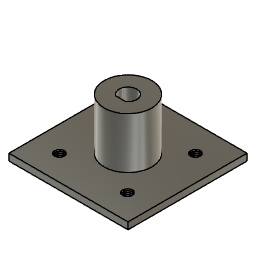
20mm_shaft_extension (Autodesk Fusion 360 design; units mm, degrees)
Autodesk Fusion 360 part; units mm, degrees
sketch "Sketch1" plane through (0, 0, 0) normal (0, 0, 1) x (1, 0, 0)
  line L0 (0, 0) -> (35, 0)
  line L1 (35, 0) -> (35, 35)
  line L2 (35, 35) -> (0, 35)
  line L3 (0, 35) -> (0, 0)
  dimension "d1" = 35
  dimension "d2" = 35
  constraint horizontal L0
  constraint vertical L1
  constraint horizontal L2
  constraint vertical L3
  constraint coincident L0.start L3.end
  measures "d1" distance of L0.start L0.end
  measures "d2" distance of L0.start L2.end
extrude "Extrude1" add sketch "Sketch1" along normal blind 2
sketch "Sketch2" plane through (0, 0, 2) normal (0, 0, 1) x (-1, 0, 0)
  line L0 (0, -35) -> (0, 0)
  line L1 (0, 0) -> (-35, 0)
  line L2 (-35, 0) -> (-35, -35)
  line L3 (-35, -35) -> (0, -35)
  circle A0 centre (-7.5, -27.5) radius 1.5
  circle A1 centre (-27.5, -27.5) radius 1.5
  circle A2 centre (-7.5, -7.5) radius 1.5
  circle A3 centre (-27.5, -7.5) radius 1.5
  dimension "d6" = 3
  dimension "d7" = 3
  dimension "d8" = 3
  dimension "d9" = 3
  dimension "d30" = 20
  dimension "d31" = 20
  dimension "d32" = 20
  dimension "d33" = 20
  dimension "d34" = 7.5
  dimension "d35" = 7.5
  measures "d6" diameter of A0
  measures "d7" diameter of A1
  measures "d8" diameter of A2
  measures "d9" diameter of A3
  measures "d30" distance of A0.centre A1.centre
  measures "d31" distance of A2.centre A3.centre
  measures "d32" distance of A0.centre A2.centre
  measures "d33" distance of A1.centre A3.centre
  measures "d34" distance of L0 A0.centre
  measures "d35" distance of L1 A2.centre
hole "Hole1" at (7.5, 27.5, 2) at (27.5, 27.5, 2) at (27.5, 7.5, 2) at (7.5, 7.5, 2) direction (0, 0, -1) diameter 2.529 depth 2 tip angle 118
thread "Thread1" "ISO Metric profile 3.0 M3x0.5 M3x0.5 6H" major diameter 3.086 minor diameter 2.529 pitch 0.5 angle 60 modelled right hand crest width 0.1368 on face at (27.6259, 6.2418, 1.3333) crest through (28.7645, 7.5, 1.875) on face at (7.6259, 26.2418, 1.3333) crest through (8.7645, 27.5, 1.875) on face at (7.6259, 6.2418, 1.3333) crest through (8.7645, 7.5, 1.875) on face at (27.6259, 26.2418, 1.3333) crest through (28.7645, 27.5, 1.875)
sketch "Sketch3" plane through (0, 0, 2) normal (0, 0, 1) x (-1, 0, 0)
  spline S0 degree 3 poles (-28.4581, -8.3252) (-28.5802, -8.2112) (-28.6784, -8.074) (-28.8207, -7.764) (-28.8611, -7.593) (-28.8757, -7.2382) (-28.8471, -7.0577) (-28.7212, -6.7109) (-28.6226, -6.5488) (-28.4156, -6.3208) (-28.3244, -6.2423) (-28.1232, -6.1071) (-28.0136, -6.0514) (-27.8985, -6.0094) knots 0 0 0 0 0.050111 0.050111 0.102261 0.102261 0.15645 0.15645 0.212677 0.212677 0.24852 0.24852 0.285143 0.285143 0.285143 0.285143
  arc A0 (-27.1015, -6.0094) -> (-27.8985, -6.0094) centre (-27.5, -7.5) ccw
  spline S1 degree 3 poles (-27.1015, -6.0094) (-26.9166, -6.0769) (-26.7465, -6.1793) (-26.4611, -6.4399) (-26.3468, -6.5935) (-26.1876, -6.9304) (-26.1419, -7.1092) (-26.1233, -7.4674) (-26.148, -7.6432) (-26.241, -7.9082) (-26.2875, -8.0028) (-26.401, -8.1765) (-26.467, -8.2553) (-26.5419, -8.3252) knots 0 0 0 0 0.059039 0.059039 0.116033 0.116033 0.170983 0.170983 0.223888 0.223888 0.255505 0.255505 0.286347 0.286347 0.286347 0.286347
  arc A1 (-28.4581, -8.3252) -> (-26.5419, -8.3252) centre (-27.5, -7.5) ccw
  spline S2 degree 3 poles (-8.4581, -28.3252) (-8.5802, -28.2112) (-8.6784, -28.074) (-8.8207, -27.764) (-8.8611, -27.593) (-8.8757, -27.2382) (-8.8471, -27.0577) (-8.7212, -26.7109) (-8.6226, -26.5488) (-8.4156, -26.3208) (-8.3244, -26.2423) (-8.1232, -26.1071) (-8.0136, -26.0514) (-7.8985, -26.0094) knots 0 0 0 0 0.050111 0.050111 0.102261 0.102261 0.15645 0.15645 0.212677 0.212677 0.24852 0.24852 0.285143 0.285143 0.285143 0.285143
  arc A2 (-7.1015, -26.0094) -> (-7.8985, -26.0094) centre (-7.5, -27.5) ccw
  spline S3 degree 3 poles (-7.1015, -26.0094) (-6.9166, -26.0769) (-6.7465, -26.1793) (-6.4611, -26.4399) (-6.3468, -26.5935) (-6.1876, -26.9304) (-6.1419, -27.1092) (-6.1233, -27.4674) (-6.148, -27.6432) (-6.241, -27.9082) (-6.2875, -28.0028) (-6.401, -28.1765) (-6.467, -28.2553) (-6.5419, -28.3252) knots 0 0 0 0 0.059039 0.059039 0.116033 0.116033 0.170983 0.170983 0.223888 0.223888 0.255505 0.255505 0.286347 0.286347 0.286347 0.286347
  arc A3 (-8.4581, -28.3252) -> (-6.5419, -28.3252) centre (-7.5, -27.5) ccw
  spline S4 degree 3 poles (-28.4581, -28.3252) (-28.5802, -28.2112) (-28.6784, -28.074) (-28.8207, -27.764) (-28.8611, -27.593) (-28.8757, -27.2382) (-28.8471, -27.0577) (-28.7212, -26.7109) (-28.6226, -26.5488) (-28.4156, -26.3208) (-28.3244, -26.2423) (-28.1232, -26.1071) (-28.0136, -26.0514) (-27.8985, -26.0094) knots 0 0 0 0 0.050111 0.050111 0.102261 0.102261 0.15645 0.15645 0.212677 0.212677 0.24852 0.24852 0.285143 0.285143 0.285143 0.285143
  arc A4 (-27.1015, -26.0094) -> (-27.8985, -26.0094) centre (-27.5, -27.5) ccw
  spline S5 degree 3 poles (-27.1015, -26.0094) (-26.9166, -26.0769) (-26.7465, -26.1793) (-26.4611, -26.4399) (-26.3468, -26.5935) (-26.1876, -26.9304) (-26.1419, -27.1092) (-26.1233, -27.4674) (-26.148, -27.6432) (-26.241, -27.9082) (-26.2875, -28.0028) (-26.401, -28.1765) (-26.467, -28.2553) (-26.5419, -28.3252) knots 0 0 0 0 0.059039 0.059039 0.116033 0.116033 0.170983 0.170983 0.223888 0.223888 0.255505 0.255505 0.286347 0.286347 0.286347 0.286347
  arc A5 (-28.4581, -28.3252) -> (-26.5419, -28.3252) centre (-27.5, -27.5) ccw
  spline S6 degree 3 poles (-8.4581, -8.3252) (-8.5802, -8.2112) (-8.6784, -8.074) (-8.8207, -7.764) (-8.8611, -7.593) (-8.8757, -7.2382) (-8.8471, -7.0577) (-8.7212, -6.7109) (-8.6226, -6.5488) (-8.4156, -6.3208) (-8.3244, -6.2423) (-8.1232, -6.1071) (-8.0136, -6.0514) (-7.8985, -6.0094) knots 0 0 0 0 0.050111 0.050111 0.102261 0.102261 0.15645 0.15645 0.212677 0.212677 0.24852 0.24852 0.285143 0.285143 0.285143 0.285143
  arc A6 (-7.1015, -6.0094) -> (-7.8985, -6.0094) centre (-7.5, -7.5) ccw
  spline S7 degree 3 poles (-7.1015, -6.0094) (-6.9166, -6.0769) (-6.7465, -6.1793) (-6.4611, -6.4399) (-6.3468, -6.5935) (-6.1876, -6.9304) (-6.1419, -7.1092) (-6.1233, -7.4674) (-6.148, -7.6432) (-6.241, -7.9082) (-6.2875, -8.0028) (-6.401, -8.1765) (-6.467, -8.2553) (-6.5419, -8.3252) knots 0 0 0 0 0.059039 0.059039 0.116033 0.116033 0.170983 0.170983 0.223888 0.223888 0.255505 0.255505 0.286347 0.286347 0.286347 0.286347
  arc A7 (-8.4581, -8.3252) -> (-6.5419, -8.3252) centre (-7.5, -7.5) ccw
  line L0 (0, -35) -> (0, 0)
  line L1 (0, 0) -> (-35, 0)
  line L2 (-35, 0) -> (-35, -35)
  line L3 (-35, -35) -> (0, -35)
  circle A8 centre (-17.5, -17.5) radius 12
  dimension "d15" = 24
  dimension "d16" = 17.5
  dimension "d17" = 17.5
  measures "d15" diameter of A8
  measures "d16" distance of L2 A8.centre
  measures "d17" distance of L3 A8.centre
extrude "Extrude2" add sketch "Sketch3" along normal blind 20 contours A8
sketch "Sketch4" plane through (0, 0, 22) normal (0, 0, 1) x (-1, 0, 0)
  circle A0 centre (-17.5, -17.5) radius 12
  circle A1 centre (-17.5, -17.5) radius 7
  dimension "d20" = 14
  constraint concentric A0 A1
  measures "d20" diameter of A1
extrude "Extrude3" add sketch "Sketch4" along normal blind 20 contours A1
sketch "Sketch5" plane through (0, 0, 42) normal (0, 0, 1) x (-1, 0, 0)
  circle A0 centre (-17.5, -17.5) radius 7
  line L0 (-16.0593, -15.3057) -> (-18.9407, -15.3057)
  arc A1 (-18.9407, -15.3057) -> (-16.0593, -15.3057) centre (-17.5, -17.5) ccw
  dimension "d23" = 5.25
  constraint concentric A0 A1
  constraint horizontal L0
  measures "d23" diameter of A1
extrude "Extrude4" cut sketch "Sketch5" against normal blind 39 contours L0 A1
extrude "Extrude5" cut 1 faces at (7.2113, 18.0962, 22) along direction (0, 0, -1) blind 20
extrude "Extrude6" cut 1 faces at (17.3256, 13.7103, 42) along direction (0, 0, -1) blind 25
